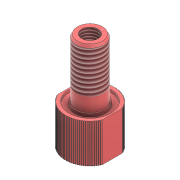
# Autodesk Inventor part: Cuerpo_interruptor_BlueRobotics
Saved by Autodesk Inventor 2022.3 (Build 263350000, 350)
## iProperties
Created: 2023-07-17
Part Number: Cuerpo_interruptor_BlueRobotics
Material: Genérico
Document SubType Name: Modeling
Designer: Usuario
Density: 1 g/cm^3
Appearance: Valor por defecto
Author: Usuario
Autodesk Inventor part; units mm, degrees
ref_plane "YZ Plane" through (0, 0, 0) normal (1, 0, 0) x (0, 1, 0)
ref_plane "XZ Plane" through (0, 0, 0) normal (0, 1, 0) x (-1, 0, 0)
ref_plane "XY Plane" through (0, 0, 0) normal (0, 0, 1) x (1, 0, 0)
sketch "Boceto1" plane through (0, 0, 0) normal (0, 1, 0) x (-1, 0, 0)
  arc A0 (-1.4277, -8.7155) -> (-1.3354, -8.7302) centre (-1.3788, -8.7053) ccw
  arc A1 (-0.8776, -8.788) -> (-1.3354, -8.7302) centre (-1.1186, -8.8546) ccw
  arc A2 (-0.8776, -8.788) -> (-0.7846, -8.7968) centre (-0.8295, -8.7747) ccw
  arc A3 (-0.3241, -8.8258) -> (-0.7846, -8.7968) centre (-0.5604, -8.9074) ccw
  arc A4 (-0.3241, -8.8258) -> (-0.2307, -8.8287) centre (-0.2768, -8.8094) ccw
  arc A5 (0.2307, -8.8287) -> (-0.2307, -8.8287) centre (0, -8.925) ccw
  arc A6 (0.2307, -8.8287) -> (0.3241, -8.8258) centre (0.2768, -8.8094) ccw
  arc A7 (0.7846, -8.7968) -> (0.3241, -8.8258) centre (0.5604, -8.9074) ccw
  arc A8 (0.7846, -8.7968) -> (0.8776, -8.788) centre (0.8295, -8.7747) ccw
  arc A9 (1.3354, -8.7302) -> (0.8776, -8.788) centre (1.1186, -8.8546) ccw
  arc A10 (1.3354, -8.7302) -> (1.4277, -8.7155) centre (1.3788, -8.7053) ccw
  arc A11 (1.881, -8.6291) -> (1.4277, -8.7155) centre (1.6724, -8.7669) ccw
  arc A12 (1.881, -8.6291) -> (1.9721, -8.6087) centre (1.9227, -8.6015) ccw
  arc A13 (2.4191, -8.494) -> (1.9721, -8.6087) centre (2.2196, -8.6446) ccw
  arc A14 (2.4191, -8.494) -> (2.5088, -8.4679) centre (2.459, -8.4638) ccw
  arc A15 (2.9476, -8.3253) -> (2.5088, -8.4679) centre (2.758, -8.4882) ccw
  arc A16 (2.9476, -8.3253) -> (3.0356, -8.2936) centre (2.9856, -8.2927) ccw
  arc A17 (3.4646, -8.1238) -> (3.0356, -8.2936) centre (3.2855, -8.2983) ccw
  arc A18 (3.4646, -8.1238) -> (3.5503, -8.0867) centre (3.5004, -8.0889) ccw
  arc A19 (3.9678, -7.8902) -> (3.5503, -8.0867) centre (3.8001, -8.0756) ccw
  arc A20 (3.9678, -7.8902) -> (4.0511, -7.8478) centre (4.0014, -7.8531) ccw
  arc A21 (4.4554, -7.6255) -> (4.0511, -7.8478) centre (4.2997, -7.821) ccw
  arc A22 (4.4554, -7.6255) -> (4.5359, -7.5779) centre (4.4866, -7.5864) ccw
  arc A23 (4.9254, -7.3307) -> (4.5359, -7.5779) centre (4.7823, -7.5356) ccw
  arc A24 (4.9254, -7.3307) -> (5.0027, -7.2782) centre (4.9541, -7.2897) ccw
  arc A25 (5.376, -7.007) -> (5.0027, -7.2782) centre (5.246, -7.2205) ccw
  arc A26 (5.376, -7.007) -> (5.4499, -6.9497) centre (5.402, -6.9643) ccw
  arc A27 (5.8054, -6.6556) -> (5.4499, -6.9497) centre (5.689, -6.8768) ccw
  arc A28 (5.8054, -6.6556) -> (5.8755, -6.5938) centre (5.8287, -6.6113) ccw
  arc A29 (6.2118, -6.2779) -> (5.8755, -6.5938) centre (6.1096, -6.506) ccw
  arc A30 (6.2118, -6.2779) -> (6.2779, -6.2118) centre (6.2323, -6.2323) ccw
  arc A31 (6.5938, -5.8755) -> (6.2779, -6.2118) centre (6.506, -6.1096) ccw
  arc A32 (6.5938, -5.8755) -> (6.6556, -5.8054) centre (6.6113, -5.8287) ccw
  arc A33 (6.9497, -5.4499) -> (6.6556, -5.8054) centre (6.8768, -5.689) ccw
  arc A34 (6.9497, -5.4499) -> (7.007, -5.376) centre (6.9643, -5.402) ccw
  arc A35 (7.2782, -5.0027) -> (7.007, -5.376) centre (7.2205, -5.246) ccw
  arc A36 (7.2782, -5.0027) -> (7.3307, -4.9254) centre (7.2897, -4.9541) ccw
  arc A37 (7.5779, -4.5359) -> (7.3307, -4.9254) centre (7.5356, -4.7823) ccw
  arc A38 (7.5779, -4.5359) -> (7.6255, -4.4554) centre (7.5864, -4.4866) ccw
  arc A39 (7.8478, -4.0511) -> (7.6255, -4.4554) centre (7.821, -4.2997) ccw
  arc A40 (7.8478, -4.0511) -> (7.8902, -3.9678) centre (7.8531, -4.0014) ccw
  arc A41 (8.0867, -3.5503) -> (7.8902, -3.9678) centre (8.0756, -3.8001) ccw
  arc A42 (8.0867, -3.5503) -> (8.1238, -3.4646) centre (8.0889, -3.5004) ccw
  arc A43 (8.2936, -3.0356) -> (8.1238, -3.4646) centre (8.2983, -3.2855) ccw
  arc A44 (8.2936, -3.0356) -> (8.3253, -2.9476) centre (8.2927, -2.9856) ccw
  arc A45 (8.4679, -2.5088) -> (8.3253, -2.9476) centre (8.4882, -2.758) ccw
  arc A46 (8.4679, -2.5088) -> (8.494, -2.4191) centre (8.4638, -2.459) ccw
  arc A47 (8.6087, -1.9721) -> (8.494, -2.4191) centre (8.6446, -2.2196) ccw
  arc A48 (8.6087, -1.9721) -> (8.6291, -1.881) centre (8.6015, -1.9227) ccw
  arc A49 (8.7155, -1.4277) -> (8.6291, -1.881) centre (8.7669, -1.6724) ccw
  arc A50 (8.7155, -1.4277) -> (8.7302, -1.3354) centre (8.7053, -1.3788) ccw
  arc A51 (8.788, -0.8776) -> (8.7302, -1.3354) centre (8.8546, -1.1186) ccw
  arc A52 (8.788, -0.8776) -> (8.7968, -0.7846) centre (8.7747, -0.8295) ccw
  arc A53 (8.8258, -0.3241) -> (8.7968, -0.7846) centre (8.9074, -0.5604) ccw
  arc A54 (8.8258, -0.3241) -> (8.8287, -0.2307) centre (8.8094, -0.2768) ccw
  arc A55 (8.8287, 0.2307) -> (8.8287, -0.2307) centre (8.925, 0) ccw
  arc A56 (8.8287, 0.2307) -> (8.8258, 0.3241) centre (8.8094, 0.2768) ccw
  arc A57 (8.7968, 0.7846) -> (8.8258, 0.3241) centre (8.9074, 0.5604) ccw
  arc A58 (8.7968, 0.7846) -> (8.788, 0.8776) centre (8.7747, 0.8295) ccw
  arc A59 (8.7302, 1.3354) -> (8.788, 0.8776) centre (8.8546, 1.1186) ccw
  arc A60 (8.7302, 1.3354) -> (8.7155, 1.4277) centre (8.7053, 1.3788) ccw
  arc A61 (8.6291, 1.881) -> (8.7155, 1.4277) centre (8.7669, 1.6724) ccw
  arc A62 (8.6291, 1.881) -> (8.6087, 1.9721) centre (8.6015, 1.9227) ccw
  arc A63 (8.494, 2.4191) -> (8.6087, 1.9721) centre (8.6446, 2.2196) ccw
  arc A64 (8.494, 2.4191) -> (8.4679, 2.5088) centre (8.4638, 2.459) ccw
  arc A65 (8.3253, 2.9476) -> (8.4679, 2.5088) centre (8.4882, 2.758) ccw
  arc A66 (8.3253, 2.9476) -> (8.2936, 3.0356) centre (8.2927, 2.9856) ccw
  arc A67 (8.1238, 3.4646) -> (8.2936, 3.0356) centre (8.2983, 3.2855) ccw
  arc A68 (8.1238, 3.4646) -> (8.0867, 3.5503) centre (8.0889, 3.5004) ccw
  arc A69 (7.8902, 3.9678) -> (8.0867, 3.5503) centre (8.0756, 3.8001) ccw
  arc A70 (7.8902, 3.9678) -> (7.8478, 4.0511) centre (7.8531, 4.0014) ccw
  arc A71 (7.6255, 4.4554) -> (7.8478, 4.0511) centre (7.821, 4.2997) ccw
  arc A72 (7.6255, 4.4554) -> (7.5779, 4.5359) centre (7.5864, 4.4866) ccw
  arc A73 (7.3307, 4.9254) -> (7.5779, 4.5359) centre (7.5356, 4.7823) ccw
  arc A74 (7.3307, 4.9254) -> (7.2782, 5.0027) centre (7.2897, 4.9541) ccw
  arc A75 (7.007, 5.376) -> (7.2782, 5.0027) centre (7.2205, 5.246) ccw
  arc A76 (7.007, 5.376) -> (6.9497, 5.4499) centre (6.9643, 5.402) ccw
  arc A77 (6.6556, 5.8054) -> (6.9497, 5.4499) centre (6.8768, 5.689) ccw
  arc A78 (6.6556, 5.8054) -> (6.5938, 5.8755) centre (6.6113, 5.8287) ccw
  arc A79 (6.2779, 6.2118) -> (6.5938, 5.8755) centre (6.506, 6.1096) ccw
  arc A80 (6.2779, 6.2118) -> (6.2118, 6.2779) centre (6.2323, 6.2323) ccw
  arc A81 (5.8755, 6.5938) -> (6.2118, 6.2779) centre (6.1096, 6.506) ccw
  arc A82 (5.8755, 6.5938) -> (5.8054, 6.6556) centre (5.8287, 6.6113) ccw
  arc A83 (5.4499, 6.9497) -> (5.8054, 6.6556) centre (5.689, 6.8768) ccw
  arc A84 (5.4499, 6.9497) -> (5.376, 7.007) centre (5.402, 6.9643) ccw
  arc A85 (5.0027, 7.2782) -> (5.376, 7.007) centre (5.246, 7.2205) ccw
  arc A86 (5.0027, 7.2782) -> (4.9254, 7.3307) centre (4.9541, 7.2897) ccw
  arc A87 (4.5359, 7.5779) -> (4.9254, 7.3307) centre (4.7823, 7.5356) ccw
  arc A88 (4.5359, 7.5779) -> (4.4554, 7.6255) centre (4.4866, 7.5864) ccw
  arc A89 (4.0511, 7.8478) -> (4.4554, 7.6255) centre (4.2997, 7.821) ccw
  arc A90 (4.0511, 7.8478) -> (3.9678, 7.8902) centre (4.0014, 7.8531) ccw
  arc A91 (3.5503, 8.0867) -> (3.9678, 7.8902) centre (3.8001, 8.0756) ccw
  arc A92 (3.5503, 8.0867) -> (3.4646, 8.1238) centre (3.5004, 8.0889) ccw
  arc A93 (3.0356, 8.2936) -> (3.4646, 8.1238) centre (3.2855, 8.2983) ccw
  arc A94 (3.0356, 8.2936) -> (2.9476, 8.3253) centre (2.9856, 8.2927) ccw
  arc A95 (2.5088, 8.4679) -> (2.9476, 8.3253) centre (2.758, 8.4882) ccw
  arc A96 (2.5088, 8.4679) -> (2.4191, 8.494) centre (2.459, 8.4638) ccw
  arc A97 (1.9721, 8.6087) -> (2.4191, 8.494) centre (2.2196, 8.6446) ccw
  arc A98 (1.9721, 8.6087) -> (1.881, 8.6291) centre (1.9227, 8.6015) ccw
  arc A99 (1.4277, 8.7155) -> (1.881, 8.6291) centre (1.6724, 8.7669) ccw
  arc A100 (1.4277, 8.7155) -> (1.3354, 8.7302) centre (1.3788, 8.7053) ccw
  arc A101 (0.8776, 8.788) -> (1.3354, 8.7302) centre (1.1186, 8.8546) ccw
  arc A102 (0.8776, 8.788) -> (0.7846, 8.7968) centre (0.8295, 8.7747) ccw
  arc A103 (0.3241, 8.8258) -> (0.7846, 8.7968) centre (0.5604, 8.9074) ccw
  arc A104 (0.3241, 8.8258) -> (0.2307, 8.8287) centre (0.2768, 8.8094) ccw
  arc A105 (-0.2307, 8.8287) -> (0.2307, 8.8287) centre (0, 8.925) ccw
  arc A106 (-0.2307, 8.8287) -> (-0.3241, 8.8258) centre (-0.2768, 8.8094) ccw
  arc A107 (-0.7846, 8.7968) -> (-0.3241, 8.8258) centre (-0.5604, 8.9074) ccw
  arc A108 (-0.7846, 8.7968) -> (-0.8776, 8.788) centre (-0.8295, 8.7747) ccw
  arc A109 (-1.3354, 8.7302) -> (-0.8776, 8.788) centre (-1.1186, 8.8546) ccw
  arc A110 (-1.3354, 8.7302) -> (-1.4277, 8.7155) centre (-1.3788, 8.7053) ccw
  arc A111 (-1.881, 8.6291) -> (-1.4277, 8.7155) centre (-1.6724, 8.7669) ccw
  arc A112 (-1.881, 8.6291) -> (-1.9721, 8.6087) centre (-1.9227, 8.6015) ccw
  arc A113 (-2.4191, 8.494) -> (-1.9721, 8.6087) centre (-2.2196, 8.6446) ccw
  arc A114 (-2.4191, 8.494) -> (-2.5088, 8.4679) centre (-2.459, 8.4638) ccw
  arc A115 (-2.9476, 8.3253) -> (-2.5088, 8.4679) centre (-2.758, 8.4882) ccw
  arc A116 (-2.9476, 8.3253) -> (-3.0356, 8.2936) centre (-2.9856, 8.2927) ccw
  arc A117 (-3.4646, 8.1238) -> (-3.0356, 8.2936) centre (-3.2855, 8.2983) ccw
  arc A118 (-3.4646, 8.1238) -> (-3.5503, 8.0867) centre (-3.5004, 8.0889) ccw
  arc A119 (-3.9678, 7.8902) -> (-3.5503, 8.0867) centre (-3.8001, 8.0756) ccw
  arc A120 (-3.9678, 7.8902) -> (-4.0511, 7.8478) centre (-4.0014, 7.8531) ccw
  arc A121 (-4.4554, 7.6255) -> (-4.0511, 7.8478) centre (-4.2997, 7.821) ccw
  arc A122 (-4.4554, 7.6255) -> (-4.5359, 7.5779) centre (-4.4866, 7.5864) ccw
  arc A123 (-4.9254, 7.3307) -> (-4.5359, 7.5779) centre (-4.7823, 7.5356) ccw
  arc A124 (-4.9254, 7.3307) -> (-5.0027, 7.2782) centre (-4.9541, 7.2897) ccw
  arc A125 (-5.376, 7.007) -> (-5.0027, 7.2782) centre (-5.246, 7.2205) ccw
  arc A126 (-5.376, 7.007) -> (-5.4499, 6.9497) centre (-5.402, 6.9643) ccw
  arc A127 (-5.8054, 6.6556) -> (-5.4499, 6.9497) centre (-5.689, 6.8768) ccw
  arc A128 (-5.8054, 6.6556) -> (-5.8755, 6.5938) centre (-5.8287, 6.6113) ccw
  arc A129 (-6.2118, 6.2779) -> (-5.8755, 6.5938) centre (-6.1096, 6.506) ccw
  arc A130 (-6.2118, 6.2779) -> (-6.2779, 6.2118) centre (-6.2323, 6.2323) ccw
  arc A131 (-6.5938, 5.8755) -> (-6.2779, 6.2118) centre (-6.506, 6.1096) ccw
  arc A132 (-6.5938, 5.8755) -> (-6.6556, 5.8054) centre (-6.6113, 5.8287) ccw
  arc A133 (-6.9497, 5.4499) -> (-6.6556, 5.8054) centre (-6.8768, 5.689) ccw
  arc A134 (-6.9497, 5.4499) -> (-7.007, 5.376) centre (-6.9643, 5.402) ccw
  arc A135 (-7.2782, 5.0027) -> (-7.007, 5.376) centre (-7.2205, 5.246) ccw
  arc A136 (-7.2782, 5.0027) -> (-7.3307, 4.9254) centre (-7.2897, 4.9541) ccw
  arc A137 (-7.5779, 4.5359) -> (-7.3307, 4.9254) centre (-7.5356, 4.7823) ccw
  arc A138 (-7.5779, 4.5359) -> (-7.6255, 4.4554) centre (-7.5864, 4.4866) ccw
  arc A139 (-7.8478, 4.0511) -> (-7.6255, 4.4554) centre (-7.821, 4.2997) ccw
  arc A140 (-7.8478, 4.0511) -> (-7.8902, 3.9678) centre (-7.8531, 4.0014) ccw
  arc A141 (-8.0867, 3.5503) -> (-7.8902, 3.9678) centre (-8.0756, 3.8001) ccw
  arc A142 (-8.0867, 3.5503) -> (-8.1238, 3.4646) centre (-8.0889, 3.5004) ccw
  arc A143 (-8.2936, 3.0356) -> (-8.1238, 3.4646) centre (-8.2983, 3.2855) ccw
  arc A144 (-8.2936, 3.0356) -> (-8.3253, 2.9476) centre (-8.2927, 2.9856) ccw
  arc A145 (-8.4679, 2.5088) -> (-8.3253, 2.9476) centre (-8.4882, 2.758) ccw
  arc A146 (-8.4679, 2.5088) -> (-8.494, 2.4191) centre (-8.4638, 2.459) ccw
  arc A147 (-8.6087, 1.9721) -> (-8.494, 2.4191) centre (-8.6446, 2.2196) ccw
  arc A148 (-8.6087, 1.9721) -> (-8.6291, 1.881) centre (-8.6015, 1.9227) ccw
  arc A149 (-8.7155, 1.4277) -> (-8.6291, 1.881) centre (-8.7669, 1.6724) ccw
  arc A150 (-8.7155, 1.4277) -> (-8.7302, 1.3354) centre (-8.7053, 1.3788) ccw
  arc A151 (-8.788, 0.8776) -> (-8.7302, 1.3354) centre (-8.8546, 1.1186) ccw
  arc A152 (-8.788, 0.8776) -> (-8.7968, 0.7846) centre (-8.7747, 0.8295) ccw
  arc A153 (-8.8258, 0.3241) -> (-8.7968, 0.7846) centre (-8.9074, 0.5604) ccw
  arc A154 (-8.8258, 0.3241) -> (-8.8287, 0.2307) centre (-8.8094, 0.2768) ccw
  arc A155 (-8.8287, -0.2307) -> (-8.8287, 0.2307) centre (-8.925, 0) ccw
  arc A156 (-8.8287, -0.2307) -> (-8.8258, -0.3241) centre (-8.8094, -0.2768) ccw
  arc A157 (-8.7968, -0.7846) -> (-8.8258, -0.3241) centre (-8.9074, -0.5604) ccw
  arc A158 (-8.7968, -0.7846) -> (-8.788, -0.8776) centre (-8.7747, -0.8295) ccw
  arc A159 (-8.7302, -1.3354) -> (-8.788, -0.8776) centre (-8.8546, -1.1186) ccw
  arc A160 (-8.7302, -1.3354) -> (-8.7155, -1.4277) centre (-8.7053, -1.3788) ccw
  arc A161 (-8.6291, -1.881) -> (-8.7155, -1.4277) centre (-8.7669, -1.6724) ccw
  arc A162 (-8.6291, -1.881) -> (-8.6087, -1.9721) centre (-8.6015, -1.9227) ccw
  arc A163 (-8.494, -2.4191) -> (-8.6087, -1.9721) centre (-8.6446, -2.2196) ccw
  arc A164 (-8.494, -2.4191) -> (-8.4679, -2.5088) centre (-8.4638, -2.459) ccw
  arc A165 (-8.3253, -2.9476) -> (-8.4679, -2.5088) centre (-8.4882, -2.758) ccw
  arc A166 (-8.3253, -2.9476) -> (-8.2936, -3.0356) centre (-8.2927, -2.9856) ccw
  arc A167 (-8.1238, -3.4646) -> (-8.2936, -3.0356) centre (-8.2983, -3.2855) ccw
  arc A168 (-8.1238, -3.4646) -> (-8.0867, -3.5503) centre (-8.0889, -3.5004) ccw
  arc A169 (-7.8902, -3.9678) -> (-8.0867, -3.5503) centre (-8.0756, -3.8001) ccw
  arc A170 (-7.8902, -3.9678) -> (-7.8478, -4.0511) centre (-7.8531, -4.0014) ccw
  arc A171 (-7.6255, -4.4554) -> (-7.8478, -4.0511) centre (-7.821, -4.2997) ccw
  arc A172 (-7.6255, -4.4554) -> (-7.5779, -4.5359) centre (-7.5864, -4.4866) ccw
  arc A173 (-7.3307, -4.9254) -> (-7.5779, -4.5359) centre (-7.5356, -4.7823) ccw
  arc A174 (-7.3307, -4.9254) -> (-7.2782, -5.0027) centre (-7.2897, -4.9541) ccw
  arc A175 (-7.007, -5.376) -> (-7.2782, -5.0027) centre (-7.2205, -5.246) ccw
  arc A176 (-7.007, -5.376) -> (-6.9497, -5.4499) centre (-6.9643, -5.402) ccw
  arc A177 (-6.6556, -5.8054) -> (-6.9497, -5.4499) centre (-6.8768, -5.689) ccw
  arc A178 (-6.6556, -5.8054) -> (-6.5938, -5.8755) centre (-6.6113, -5.8287) ccw
  arc A179 (-6.2779, -6.2118) -> (-6.5938, -5.8755) centre (-6.506, -6.1096) ccw
  arc A180 (-6.2779, -6.2118) -> (-6.2118, -6.2779) centre (-6.2323, -6.2323) ccw
  arc A181 (-5.8755, -6.5938) -> (-6.2118, -6.2779) centre (-6.1096, -6.506) ccw
  arc A182 (-5.8755, -6.5938) -> (-5.8054, -6.6556) centre (-5.8287, -6.6113) ccw
  arc A183 (-5.4499, -6.9497) -> (-5.8054, -6.6556) centre (-5.689, -6.8768) ccw
  arc A184 (-5.4499, -6.9497) -> (-5.376, -7.007) centre (-5.402, -6.9643) ccw
  arc A185 (-5.0027, -7.2782) -> (-5.376, -7.007) centre (-5.246, -7.2205) ccw
  arc A186 (-5.0027, -7.2782) -> (-4.9254, -7.3307) centre (-4.9541, -7.2897) ccw
  arc A187 (-4.5359, -7.5779) -> (-4.9254, -7.3307) centre (-4.7823, -7.5356) ccw
  arc A188 (-4.5359, -7.5779) -> (-4.4554, -7.6255) centre (-4.4866, -7.5864) ccw
  arc A189 (-4.0511, -7.8478) -> (-4.4554, -7.6255) centre (-4.2997, -7.821) ccw
  arc A190 (-4.0511, -7.8478) -> (-3.9678, -7.8902) centre (-4.0014, -7.8531) ccw
  arc A191 (-3.5503, -8.0867) -> (-3.9678, -7.8902) centre (-3.8001, -8.0756) ccw
  arc A192 (-3.5503, -8.0867) -> (-3.4646, -8.1238) centre (-3.5004, -8.0889) ccw
  arc A193 (-3.0356, -8.2936) -> (-3.4646, -8.1238) centre (-3.2855, -8.2983) ccw
  arc A194 (-3.0356, -8.2936) -> (-2.9476, -8.3253) centre (-2.9856, -8.2927) ccw
  arc A195 (-2.5088, -8.4679) -> (-2.9476, -8.3253) centre (-2.758, -8.4882) ccw
  arc A196 (-2.5088, -8.4679) -> (-2.4191, -8.494) centre (-2.459, -8.4638) ccw
  arc A197 (-1.9721, -8.6087) -> (-2.4191, -8.494) centre (-2.2196, -8.6446) ccw
  arc A198 (-1.9721, -8.6087) -> (-1.881, -8.6291) centre (-1.9227, -8.6015) ccw
  arc A199 (-1.4277, -8.7155) -> (-1.881, -8.6291) centre (-1.6724, -8.7669) ccw
  point P0 (0, 0)
  point P1 (0, 0)
  constraints: 400 point on circle, 200 centre point
extrude "Extrusión1" add sketch "Boceto1" along normal blind 14
sketch "Boceto2" plane through (0, 14, 0) normal (0, 1, 0) x (1, 0, 0)
  line L0 (0, 0) -> (-8, 0)
  line L1 (-8, 0) -> (-8, 7.8928)
  line L2 (-8, 7.8928) -> (-10.6543, 7.8928)
  line L3 (-10.6543, 7.8928) -> (-10.6543, -7.3053)
  line L4 (-10.6543, -7.3053) -> (-8, -7.3053)
  line L5 (-8, -7.3053) -> (-8, 0)
  line L6 (0, 0) -> (8, 0)
  line L7 (8, 0) -> (8, 10.2039)
  line L8 (8, 10.2039) -> (11.046, 10.2039)
  line L9 (11.046, 10.2039) -> (11.046, -9.3421)
  line L10 (11.046, -9.3421) -> (8, -9.3421)
  line L11 (8, -9.3421) -> (8, 0)
  dimension "d2" = 8
  dimension "d3" = 8
  constraints: 24 end point, 9 perpendicular, 2 horizontal, 2 point on line, 1 collinear
  measures "d2" distance of L0.start L0.end
  measures "d3" distance of L0.start L6.end
extrude "Extrusión2" cut sketch "Boceto2" against normal blind 14
sketch "Boceto3" plane through (0, 14, 0) normal (0, 1, 0) x (1, 0, 0)
  circle A0 centre (0, 0) radius 5
  dimension "d6" = 10
  constraints: 1 centre point, 1 coincident
  measures "d6" diameter of A0
extrude "Extrusión3" add sketch "Boceto3" along normal blind 21.1
thread "Rosca1" size "M10x1.5" class "6g" standard "ANSI Metric M Profile" length 21.1 offset 5
sketch "Boceto4" plane through (0, 35.1, 0) normal (0, 1, 0) x (1, 0, 0)
  circle A0 centre (0, 0) radius 2.5
  dimension "d11" = 5
  constraints: 1 centre point, 1 coincident
  measures "d11" diameter of A0
extrude "Extrusión4" cut sketch "Boceto4" against normal through all
sketch "Boceto5" plane through (0, 0, 0) normal (0, -1, 0) x (1, 0, 0)
  circle A0 centre (0, 0) radius 5
  dimension "d14" = 10
  constraints: 1 centre point, 1 coincident
  measures "d14" diameter of A0
extrude "Extrusión5" cut sketch "Boceto5" against normal blind 12
thread "Rosca2" size "M5x0.8" class "6H" standard "ANSI Metric M Profile" length 5
sketch "Boceto6" plane through (0, 35.1, 0) normal (0, 1, 0) x (1, 0, 0)
  circle A0 centre (0, 0) radius 3
  dimension "d19" = 6
  constraints: 1 centre point, 1 coincident
  measures "d19" diameter of A0
extrude "Extrusión6" cut sketch "Boceto6" against normal blind 6.2
thread "Rosca3" size "M6x1" class "6H" standard "ANSI Metric M Profile" length 6.2
chamfer "Chaflán1" distance 0.5 angle 45 1 edges at (-2.5, 28.9, 0)
chamfer "Chaflán2" distance 0.5 distance2 1 1 edges at (-5, 35.1, 0) measured on face at (4.2558, 35.1, 0.6382)
sketch "Boceto7" plane through (0, 14, 0) normal (0, 1, 0) x (1, 0, 0)
  circle A0 centre (0, 0) radius 7.5
  circle A1 centre (0, 0) radius 5.5
  dimension "d30" = 15
  dimension "d31" = 11
  constraints: 2 centre point, 2 coincident
  measures "d30" diameter of A0
  measures "d31" diameter of A1
extrude "Extrusión7" cut sketch "Boceto7" against normal blind 1
